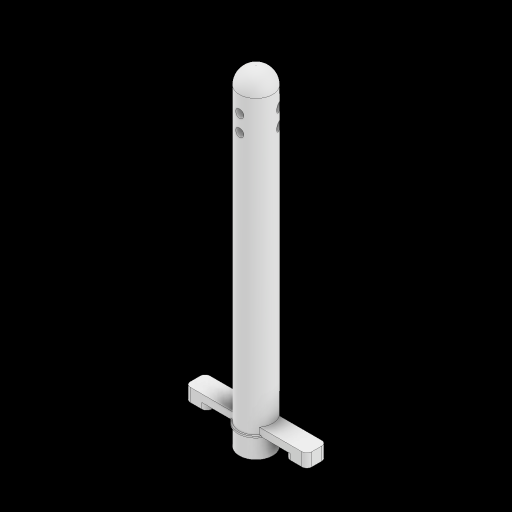
# Autodesk Inventor part: andomierz_wal
Saved by Autodesk Inventor 2024.4 (Build 284460000, 460)
## iProperties
Created: 2026-02-13
Part Number: andomierz_wal
Material: Tworzywo sztuczne ABS
Document SubType Name: Modeling
Designer: User
Density: 1.06 g/cm^3
Appearance: Gładki — biały
Mass: 64.3689 g
Surface Area: 161.595 cm^2
Volume: 64.3689 cm^3
Author: User
Autodesk Inventor part; units mm, degrees
ref_plane "YZ Plane" through (0, 0, 0) normal (1, 0, 0) x (0, 1, 0)
sketch "Szkic1" plane through (0, 0, 0) normal (0, 1, 0) x (-1, 0, 0)
  circle A0 centre (0, 0) radius 10.1
  dimension "d0" = 20.2
  constraints: 1 centre point, 1 coincident
  measures "d0" diameter of A0
extrude "Wyciągnięcie proste1" add sketch "Szkic1" along normal blind 200
ref_plane "Płaszczyzna konstrukcyjna1" through (0, 13, 0) normal (0, -1, 0) x (1, 0, 0)
sketch "Szkic2" plane through (0, 13, 0) normal (0, -1, 0) x (1, 0, 0)
  line L0 (0, 0) -> (30.4, 0)
  line L1 (0, 0) -> (30.4, 0) construction
  circle A0 centre (30.4, 0) radius 5.5
  line L2 (35.9, 0) -> (36.9, 0)
  line L3 (36.9, 0) -> (0, 0)
  line L4 (0, 0) -> (0, -6)
  line L5 (0, -6) -> (36.9, -6)
  line L6 (36.9, -6) -> (36.9, 0)
  line L7 (0, 0) -> (0, -16.4984)
  line L8 (0, 6) -> (36.9, 6)
  line L9 (36.9, 6) -> (36.9, 0)
  line L10 (0, 0) -> (-30.4, 0)
  line L11 (0, 0) -> (-30.4, 0) construction
  circle A1 centre (-30.4, 0) radius 5.5
  line L12 (-35.9, 0) -> (-36.9, 0)
  line L13 (-36.9, 0) -> (0, 0)
  line L14 (0, -6) -> (-36.9, -6)
  line L15 (0, 6) -> (-36.9, 6)
  line L16 (-36.9, 6) -> (-36.9, -6)
  line L17 (-24.9, 0) -> (-23.9, 0)
  line L18 (-23.9, 0) -> (-23.9, 6)
  line L19 (-23.9, 0) -> (-23.9, -6)
  line L20 (24.9, 0) -> (23.9, 0)
  line L21 (23.9, 0) -> (23.9, 6)
  line L22 (23.9, 0) -> (23.9, -6)
  dimension "d4" = 30.4
  dimension "d5" = 0
  dimension "d6" = 11
  dimension "d7" = 1
  dimension "d8" = 6
  dimension "d13" = 1
  dimension "d14" = 1
  constraints: 46 end point, 9 symmetric about line, 8 point on line, 4 horizontal, 4 perpendicular, 4 point on circle, 2 centre point, 2 coincident, 2 parallel, 2 vertical, 1 collinear, 1 other
  measures "d4" distance of L0.start L0.end
  measures "d5" distance between parallel lines of L0 L1
  measures "d6" diameter of A0
  measures "d7" distance of L2.start L2.end
  measures "d8" distance of L4.end L3.end
  measures "d13" distance of L17.start L17.end
  measures "d14" distance of L20.start L20.end
extrude "Wyciągnięcie proste2" add sketch "Szkic2" along normal blind 0.5 contours L10 L18 L15 L8 L21 L0 | L0 L22 L5 L4 | L4 L14 L19 L10 | L21 L8 L9 L2 A0 L0 | L0 A0 L2 L6 L5 L22 | L19 L14 L16 L12 A1 L10 | L10 A1 L12 L16 L15 L18
extrude "Wyciągnięcie proste3" add sketch "Szkic2" against normal blind 4
extrude "Wyciągnięcie proste4" add sketch "Szkic2" along normal blind 4 contours L21 L8 L9 L2 A0 L0 | L0 A0 L2 L6 L5 L22 | L19 L14 L16 L12 A1 L10 | L10 A1 L12 L16 L15 L18
fillet "Zaokrąglenie1" radius 3 8 edges at (-36.9, 13, 6) (-23.9, 10.75, 6) (-36.9, 13, -6) (-23.9, 10.75, -6) (36.9, 13, 6) (23.9, 10.75, 6) (36.9, 13, -6) (23.9, 10.75, -6)
sketch "Szkic3" plane through (0, 0, 0) normal (0, 0, 1) x (1, 0, 0)
  line L0 (10.1, 200) -> (-10.1, 200) projected
  line L1 (0, 200) -> (0, 190)
  line L2 (0, 190) -> (0, 180)
  line L3 (0, 180) -> (0, 170)
  circle A0 centre (0, 170) radius 2.45
  circle A1 centre (0, 180) radius 2.45
  point P0 (0, 0)
  dimension "d21" = 10
  dimension "d22" = 10
  dimension "d23" = 10
  dimension "d24" = 4.9
  dimension "d25" = 4.9
  constraints: 6 end point, 2 centre point, 2 coincident, 2 point on line, 1 midpoint, 1 vertical
  measures "d21" distance of L1.start L1.end
  measures "d22" distance of L1.end L2.end
  measures "d23" distance of L2.end L3.end
  measures "d24" diameter of A0
  measures "d25" diameter of A1
extrude "Wyciągnięcie proste5" cut sketch "Szkic3" along normal blind 60
pattern_circular "Szyk kołowy1" count 3 over 360 about axis through (0, 0, 0) along (0, 1, 0) of "Wyciągnięcie proste5"
fillet "Zaokrąglenie2" radius 10 1 edges at (10.1, 200, 0)
ref_plane "Płaszczyzna konstrukcyjna2" through (0, 12, 0) normal (0, -1, 0) x (1, 0, 0)
sketch "Szkic4" plane through (0, 12, 0) normal (0, -1, 0) x (1, 0, 0)
  circle A0 centre (0, 0) radius 11
  dimension "d36" = 22
  constraints: 1 centre point, 1 coincident
  measures "d36" diameter of A0
extrude "Wyciągnięcie proste6" add sketch "Szkic4" against normal blind 1
sketch "Szkic5" plane through (0, 0, 0) normal (0, -1, 0) x (1, 0, 0)
  line L0 (0, -2.829) -> (0, 0) projected
  circle A0 centre (0, 0) radius 2.6
  dimension "d39" = 5.2
  constraints: 1 centre point, 1 coincident
  measures "d39" diameter of A0
extrude "Wyciągnięcie proste7" cut sketch "Szkic5" against normal blind 10
